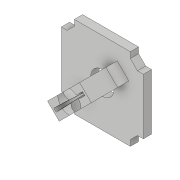
# Autodesk Inventor part: 20_Cube_Insert_Beamsplitter_Mirror45_v3
Saved by Autodesk Inventor 2019.4 (Build 234330000, 330)
## iProperties
Created: 2019-07-01
Part Number: 20_Cube_Insert_Beamsplitter_Mirror45_v3
Material: Generic
Document SubType Name: Modeling
Designer: diederichbenedict
Density: 1 g/cm^3
Appearance: Default
Author: diederichbenedict
Autodesk Inventor part; units mm, degrees
ref_plane "YZ Plane" through (0, 0, 0) normal (1, 0, 0) x (0, 1, 0)
ref_plane "XZ Plane" through (0, 0, 0) normal (0, 1, 0) x (-1, 0, 0)
ref_plane "Work Plane1" through (0, 0, 10) normal (0, 0, 1) x (1, 0, 0)
sketch "Sketch1" plane through (0, 0, 10) normal (0, 0, 1) x (1, 0, 0)
  line L0 (-4.029928, -0.353838) -> (-2.232156, 1.443934) construction
  arc A0 (-1.443934, 2.232156) -> (-2.232156, 1.443934) centre (-0.929928, 0.929928) ccw construction
  line L1 (-1.443934, 2.232156) -> (0.353838, 4.029928) construction
  line L2 (-37.829928, 42.213694) -> (-37.829928, 45.829928) construction
  line L3 (-37.829928, 45.829928) -> (-4.029928, 45.829928) construction
  line L4 (-4.029928, 45.829928) -> (-4.029928, 42.213694) construction
  line L5 (-4.029928, 4.029928) -> (0.353838, 4.029928)
  circle A1 centre (-20.929928, 20.929928) radius 17.5
  line L6 (-20.929928, 58.972273) -> (17.112417, 20.929928) construction
  line L7 (17.112417, 20.929928) -> (-20.929928, -17.112417) construction
  line L8 (-20.929928, -17.112417) -> (-58.972273, 20.929928) construction
  line L9 (-58.972273, 20.929928) -> (-20.929928, 58.972273) construction
  line L10 (-20.929928, 58.972273) -> (-20.929928, -17.112417) construction
  line L11 (17.112417, 20.929928) -> (-58.972273, 20.929928) construction
  line L12 (-20.929928, 58.972273) -> (32.870072, 58.972273) construction
  line L13 (-43.429928, 43.429928) -> (1.570072, 43.429928) construction
  line L14 (1.570072, 43.429928) -> (1.570072, -1.570072) construction
  line L15 (1.570072, -1.570072) -> (-43.429928, -1.570072) construction
  line L16 (-43.429928, -1.570072) -> (-43.429928, 43.429928) construction
  line L17 (-43.429928, 43.429928) -> (1.570072, -1.570072) construction
  line L18 (1.570072, 43.429928) -> (-43.429928, -1.570072) construction
  line L19 (-43.429928, 5.387583) -> (-43.429928, 36.472273)
  line L20 (-43.429928, 36.472273) -> (-36.472273, 43.429928)
  line L21 (-36.472273, 43.429928) -> (-5.387583, 43.429928)
  line L22 (-5.387583, 43.429928) -> (1.570072, 36.472273)
  line L23 (1.570072, 36.472273) -> (1.570072, 5.387583)
  line L24 (1.570072, 5.387583) -> (-5.387583, -1.570072)
  line L25 (-5.387583, -1.570072) -> (-36.472273, -1.570072)
  line L26 (-36.472273, -1.570072) -> (-43.429928, 5.387583)
  line L27 (-4.029928, 42.213694) -> (-37.829928, 42.213694)
  line L28 (-4.029928, -0.353838) -> (-4.029928, 4.029928)
  circle A2 centre (-20.929928, 20.929928) radius 7.04172
  point P0 (-37.829928, 4.029928)
  dimension "d18" = 53.8
  dimension "d19" = 45
  dimension "d20" = 53.8
  dimension "d21" = 45
  dimension "d22" = 45
  constraints: 42 end point, 15 point on line, 5 midpoint, 4 parallel, 3 perpendicular, 2 horizontal, 1 centre point, 1 coincident, 1 equal length
  measures "d18" distance of L6.start L6.end
  measures "d19" angle of L6 L12
  measures "d20" distance of L6.end L7.end
  measures "d21" distance of L14.end L15.end
  measures "d22" distance of L13.end L14.end
extrude "Extrusion1" add sketch "Sketch1" along normal blind 5 contours L28 L24 L25 L26 L19 L20 L27 L22 L23 L5 | L5 L24 L28 | L27 L20 L21 L22 | A1
sketch "Sketch3" plane through (0, 0, 10) normal (0, 0, -1) x (-1, 0, 0)
  line L0 (37.829928, -0.470072) -> (37.829928, 4.029928) construction
  line L1 (4.029928, 4.029928) -> (4.029928, -0.470072) construction
  line L2 (37.829928, -0.470072) -> (37.829928, 1.18864) construction
  line L3 (4.029928, -3.970072) -> (4.029928, -0.353838) construction
  line L4 (45.829928, 4.029928) -> (42.213694, 4.029928) construction
  line L5 (-0.353838, 4.029928) -> (-3.970072, 4.029928) construction
  line L6 (-3.970072, 37.829928) -> (-0.353838, 37.829928) construction
  line L7 (4.029928, 42.213694) -> (4.029928, 45.829928) construction
  line L8 (37.829928, 45.829928) -> (37.829928, 42.213694) construction
  line L9 (42.213694, 37.829928) -> (45.829928, 37.829928) construction
  line L10 (37.829928, 37.729928) -> (45.829928, 37.729928)
  line L11 (45.829928, 37.729928) -> (45.829928, 4.129928)
  line L12 (45.829928, 4.129928) -> (37.829928, 4.129928)
  line L13 (37.829928, 4.129928) -> (37.829928, 37.729928)
  line L14 (37.729928, 4.029928) -> (4.129928, 4.029928)
  line L15 (4.129928, 4.029928) -> (4.129928, -3.970072)
  line L16 (4.129928, -3.970072) -> (37.729928, -3.970072)
  line L17 (37.729928, -3.970072) -> (37.729928, 4.029928)
  line L18 (4.029928, 4.129928) -> (-3.970072, 4.129928)
  line L19 (-3.970072, 4.129928) -> (-3.970072, 37.729928)
  line L20 (-3.970072, 37.729928) -> (4.029928, 37.729928)
  line L21 (4.029928, 37.729928) -> (4.029928, 4.129928)
  line L22 (4.129928, 37.829928) -> (37.729928, 37.829928)
  line L23 (37.729928, 37.829928) -> (37.729928, 45.829928)
  line L24 (37.729928, 45.829928) -> (4.129928, 45.829928)
  line L25 (4.129928, 45.829928) -> (4.129928, 37.829928)
  point P0 (0, 0)
  dimension "d23" = 0.1
  dimension "d24" = 0.1
  dimension "d25" = 0.1
  dimension "d26" = 0.1
  dimension "d27" = 0.1
  constraints: 32 end point, 8 parallel, 4 horizontal, 4 perpendicular, 3 point on line
  measures "d23" distance between parallel lines of L8 L23
  measures "d24" distance between parallel lines of L7 L25
  measures "d25" distance between parallel lines of L6 L20
  measures "d26" distance between parallel lines of L5 L18
  measures "d27" distance between parallel lines of L1 L15
extrude "Extrusion3" add sketch "Sketch3" against normal up to surface (5 mm away)
sketch "Skizze12" plane through (0, 0, 10) normal (0, 0, -1) x (-1, 0, 0)
  line L0 (-0.312417, 4.129928) -> (4.129928, -0.312417)
  line L1 (4.129928, -0.312417) -> (4.129928, -3.970072)
  line L2 (4.129928, -3.970072) -> (37.729928, -3.970072) construction
  line L3 (37.729928, -3.970072) -> (37.729928, -0.312417)
  line L4 (37.729928, -0.312417) -> (42.172273, 4.129928)
  line L5 (45.829928, 4.129928) -> (42.172273, 4.129928)
  line L6 (45.829928, 37.729928) -> (45.829928, 4.129928) construction
  line L7 (42.172273, 37.729928) -> (45.829928, 37.729928)
  line L8 (42.172273, 37.729928) -> (37.729928, 42.172273)
  line L9 (37.729928, 42.172273) -> (37.729928, 45.829928)
  line L10 (37.729928, 45.829928) -> (4.129928, 45.829928) construction
  line L11 (4.129928, 45.829928) -> (4.129928, 42.172273)
  line L12 (4.129928, 42.172273) -> (-0.312417, 37.729928)
  line L13 (-3.970072, 37.729928) -> (-0.312417, 37.729928)
  line L14 (-3.970072, 4.129928) -> (-3.970072, 37.729928) construction
  line L15 (-0.312417, 4.129928) -> (-3.970072, 4.129928)
  circle A0 centre (20.929928, 20.929928) radius 7.04172 construction
  line L16 (37.929928, -4.170072) -> (3.929928, -4.170072) construction
  line L17 (3.929928, -4.170072) -> (3.929928, -0.39526)
  line L18 (3.929928, -0.39526) -> (-0.39526, 3.929928)
  line L19 (-0.39526, 3.929928) -> (-4.170072, 3.929928)
  line L20 (-4.170072, 3.929928) -> (-4.170072, 37.929928) construction
  line L21 (-4.170072, 37.929928) -> (-0.39526, 37.929928)
  line L22 (-0.39526, 37.929928) -> (3.929928, 42.255116)
  line L23 (3.929928, 42.255116) -> (3.929928, 46.029928)
  line L24 (3.929928, 46.029928) -> (37.929928, 46.029928) construction
  line L25 (37.929928, 46.029928) -> (37.929928, 42.255116)
  line L26 (37.929928, 42.255116) -> (42.255116, 37.929928)
  line L27 (42.255116, 37.929928) -> (46.029928, 37.929928)
  line L28 (46.029928, 37.929928) -> (46.029928, 3.929928) construction
  line L29 (46.029928, 3.929928) -> (42.255116, 3.929928)
  line L30 (42.255116, 3.929928) -> (37.929928, -0.39526)
  line L31 (37.929928, -0.39526) -> (37.929928, -4.170072)
  line L32 (-3.970072, 37.729928) -> (-3.970072, 37.929928)
  line L33 (37.729928, 45.829928) -> (4.129928, 45.829928)
  line L34 (4.129928, 45.829928) -> (3.929928, 45.829928)
  line L35 (37.729928, 45.829928) -> (37.929928, 45.829928)
  line L36 (45.829928, 37.729928) -> (45.829928, 37.929928)
  line L37 (45.829928, 4.129928) -> (45.829928, 3.929928)
  line L38 (37.729928, -3.970072) -> (37.929928, -3.970072)
  line L39 (4.129928, -3.970072) -> (3.929928, -3.970072)
  line L40 (-3.970072, 4.129928) -> (-3.970072, 3.929928)
  point P0 (0, 0)
  dimension "d65" = 0.2
  constraints: 48 end point, 13 point on line, 2 perpendicular, 1 vertical, 15 other
  measures "d65" distance between parallel lines of L2 L16
extrude "IM_offset" add sketch "Skizze12" against normal up to surface (5 mm away)
sketch "Sketch14" plane through (0, 0, 15) normal (0, 0, 1) x (1, 0, 0)
  circle A0 centre (-20.929928, 20.929928) radius 7.04172 construction
  line L0 (-34.200592, 14.730332) -> (-27.129524, 7.659264)
  line L1 (-7.659264, 27.129524) -> (-14.730332, 34.200592)
  line L2 (-14.730332, 34.200592) -> (-27.129524, 7.659264) construction
  line L3 (-34.200592, 14.730332) -> (-7.659264, 27.129524) construction
  line L4 (-14.730332, 34.200592) -> (12.804773, 34.200592) construction
  circle A1 centre (-20.929928, 20.929928) radius 7.04172
  line L5 (-14.730332, 34.200592) -> (-20.959337, 27.971586)
  line L6 (-27.971586, 20.959337) -> (-34.200592, 14.730332)
  line L7 (-27.129524, 7.659264) -> (-20.900519, 13.88827)
  line L8 (-13.88827, 20.900519) -> (-7.659264, 27.129524)
  arc A2 (-13.829451, 20.959337) -> (-20.959337, 27.971586) centre (-20.983844, 20.815796) ccw
  arc A3 (-27.971586, 20.959337) -> (-20.900519, 13.88827) centre (-20.929928, 20.929928) ccw
  point P0 (0, 0)
  dimension "d69" = 10
  constraints: 18 end point, 10 point on circle, 5 parallel, 2 centre point, 2 midpoint, 2 perpendicular, 1 concentric, 1 horizontal, 1 point on line
  measures "d69" distance of L0.end L0.start
sketch "Sketch14 outline for Extrusion12" plane through (0, 0, 15) normal (0, 0, 1) x (1, 0, 0)
  line L0 (-27.971586, 20.959337) -> (-34.200592, 14.730332)
  arc A0 (-20.900519, 13.88827) -> (-27.971586, 20.959337) centre (-20.929928, 20.929928) cw
  line L1 (-27.129524, 7.659264) -> (-20.900519, 13.88827)
  line L2 (-34.200592, 14.730332) -> (-27.129524, 7.659264)
  line L3 (-7.659264, 27.129524) -> (-14.730332, 34.200592)
  line L4 (-14.730332, 34.200592) -> (-20.959337, 27.971586)
  arc A1 (-20.959337, 27.971586) -> (-13.88827, 20.900519) centre (-20.929928, 20.929928) cw
  line L5 (-13.88827, 20.900519) -> (-7.659264, 27.129524)
extrude "Extrusion12" add sketch "Sketch14 outline for Extrusion12" along normal blind 20
sketch "Sketch15" plane through (0, 0, 35) normal (0, 0, 1) x (1, 0, 0)
  line L0 (-34.200592, 14.730332) -> (-27.129524, 7.659264)
  line L1 (-27.129524, 7.659264) -> (-20.900519, 13.88827)
  arc A0 (-27.971586, 20.959337) -> (-20.900519, 13.88827) centre (-20.929928, 20.929928) ccw
  line L2 (-27.971586, 20.959337) -> (-34.200592, 14.730332)
  line L3 (-11.560763, 28.884879) -> (-28.884879, 11.560763)
  line L4 (-28.884879, 11.560763) -> (-30.299093, 12.974977)
  line L5 (-30.299093, 12.974977) -> (-12.974977, 30.299093)
  line L6 (-12.974977, 30.299093) -> (-11.560763, 28.884879)
  line L7 (-11.560763, 28.884879) -> (-30.299093, 12.974977) construction
  line L8 (-28.884879, 11.560763) -> (-12.974977, 30.299093) construction
  point P0 (0, 0)
  dimension "d72" = 24.5
  dimension "d73" = 2
  constraints: 12 end point, 2 midpoint, 2 parallel, 1 perpendicular
  measures "d72" distance of L3.start L3.end
  measures "d73" distance of L3.end L4.end
sketch "Sketch15 outline for Extrusion13" plane through (0, 0, 35) normal (0, 0, 1) x (1, 0, 0)
  line L0 (-11.560763, 28.884879) -> (-28.884879, 11.560763)
  line L1 (-28.884879, 11.560763) -> (-30.299093, 12.974977)
  line L2 (-30.299093, 12.974977) -> (-12.974977, 30.299093)
  line L3 (-12.974977, 30.299093) -> (-11.560763, 28.884879)
extrude "Extrusion13" cut sketch "Sketch15 outline for Extrusion13" against normal blind 20 draft -2
sketch "Sketch16" plane through (3.970072, 3.929928, 10) normal (1, 0, 0) x (0, 0, -1)
  line L0 (-5, 34) -> (-5, 0)
  line L1 (0, 0) -> (-5, 0)
  line L2 (0, 0) -> (0, 34)
  line L3 (0, 34) -> (-5, 34)
  line L4 (0, 24.04172) -> (0, 9.95828)
  ellipse E0 centre (3.636253, 17) end of major axis (205.284687, 21.982283) minor radius 4.97773 (-5, 21.761427) -> (-25, 21.221677) ccw
  line L5 (-5, 21.761427) -> (-5, 22.187932)
  ellipse E1 centre (3.636253, 17) end of major axis (-198.012181, 21.982283) minor radius 4.97773 (-5, 22.187932) -> (-25, 22.63589) ccw
  line L6 (-25, 24.041658) -> (-25, 22.63589)
  line L7 (-5, 24.041658) -> (-25, 24.041658)
  line L8 (-5, 17.029409) -> (-5, 24.041658)
  line L9 (-5, 17.029409) -> (-25, 17.029409)
  line L10 (-25, 12.778323) -> (-25, 17.029409)
  ellipse E2 centre (3.636253, 17) end of major axis (-198.012181, 21.982283) minor radius 4.97773 (-25, 12.778323) -> (-5, 12.238573) ccw
  line L11 (-5, 12.238573) -> (-5, 11.812068)
  ellipse E3 centre (3.636253, 17) end of major axis (205.284687, 21.982283) minor radius 4.97773 (-25, 11.36411) -> (-5, 11.812068) ccw
  line L12 (-25, 9.958342) -> (-25, 11.36411)
  line L13 (-5, 9.958342) -> (-25, 9.958342)
  line L14 (-5, 16.970591) -> (-5, 9.958342)
  line L15 (-5, 16.970591) -> (-25, 16.970591)
  line L16 (-25, 21.221677) -> (-25, 16.970591)
  line L17 (-5, 16.970591) -> (-25, 16.970591)
  circle A0 centre (-15.553034, 16.970591) radius 6
  point P0 (10, -3.929928)
  dimension "d76" = 12
  constraints: 1 centre point, 1 point on line, 4 other
  measures "d76" diameter of A0
extrude "Extrusion14" cut sketch "Sketch16" against normal up to surface (30.53589 mm away) contours A0 E0 E1 | E1 A0 | A0 L9 E0 | A0 L15 L9 | A0 E2 L15 | A0 E3 E2 | A0 E3
pattern_circular "Circular Pattern1" count 4 over 360 about axis through (-20.929928, 20.929928, 10) along (0, 0, 1) of "Extrusion14"
chamfer "Chamfer1" distance 4 angle 45 2 edges at (-30.6651, 11.1948, 15) (-11.1948, 30.6651, 15)
body "Solid1"
